Autodesk Inventor part; units mm, degrees
note: some values were not read from the file. Chosen so that the rebuilt part matches the saved one: direction of "Hole2".
(part 11 of 18)
  arc A17 (-107.2677, -34.3213) -> (-106.7778, -34.3555) centre (-106.9408, -33.1666) ccw
  line L749 (-108.0363, -21.6967) -> (-108.0269, -21.8841)
  line L750 (-107.9752, -22.9062) -> (-107.968, -23.049)
  line L751 (-107.6573, -29.1932) -> (-107.5403, -31.5077)
  line L752 (-107.4859, -32.5836) -> (-107.4515, -33.2651)
  arc A18 (-104.3538, -35.2232) -> (-104.2354, -35.2295) centre (-104.2317, -34.0295) ccw
  line L753 (-103.7167, -34.0438) -> (-103.7199, -34.1051)
  line L754 (-104.7061, -33.2435) -> (-104.7563, -34.1999)
  line L755 (-91.4937, -33.0969) -> (-91.4774, -33.1737)
  arc A19 (-88.1095, -35.5428) -> (-87.8105, -35.509) centre (-88.0934, -34.3429) ccw
  line L756 (-87.667, -33.5285) -> (-87.5609, -34.4691)
  line L757 (-88.6914, -33.6357) -> (-88.5844, -34.5846)
  arc A20 (-106.1926, -35.509) -> (-105.8936, -35.5428) centre (-105.9097, -34.3429) ccw
  line L758 (-105.3117, -33.6357) -> (-105.4187, -34.5846)
  line L759 (-106.3361, -33.5285) -> (-106.4422, -34.4691)
  line L760 (-102.5094, -33.0969) -> (-102.5257, -33.1737)
  arc A21 (-89.7677, -35.2295) -> (-89.6493, -35.2232) centre (-89.7714, -34.0295) ccw
  line L761 (-89.297, -33.2435) -> (-89.2467, -34.1999)
  line L762 (-90.2864, -34.0438) -> (-90.2831, -34.1051)
  arc A22 (-87.2253, -34.3555) -> (-86.7354, -34.3213) centre (-87.0623, -33.1666) ccw
  line L763 (-85.9668, -21.6967) -> (-85.9762, -21.8841)
  line L764 (-86.0279, -22.9062) -> (-86.0335, -23.0165)
  line L765 (-86.3442, -29.1624) -> (-86.4628, -31.5077)
  line L766 (-86.5172, -32.5836) -> (-86.5516, -33.2651)
  line L767 (-106.1877, -21.7539) -> (-106.1874, -21.795)
  line L768 (-106.1392, -29.1135) -> (-106.136, -29.6026)
  line L769 (-88.0087, -28.9946) -> (-87.8587, -30.5301)
  line L770 (-105.9944, -28.9946) -> (-106.1444, -30.5301)
  line L771 (-87.8154, -21.7539) -> (-87.8156, -21.795)
  line L772 (-87.8638, -29.1028) -> (-87.8671, -29.6026)
  ellipse E590 centre (-107.1928, -15.9924) end of major axis (-108.8923, -16.0353) minor radius 0.2846 (-108.3788, -15.8176) -> (-108.8923, -16.0353) ccw
  line L773 (-108.8884, -16.1889) -> (-108.8923, -16.0353)
  ellipse E591 centre (-86.8103, -15.9924) end of major axis (-85.1108, -16.0353) minor radius 0.2846 (-85.1108, -16.0353) -> (-85.6243, -15.8176) ccw
  line L774 (-85.1147, -16.1889) -> (-85.1108, -16.0353)
  ellipse E592 centre (-107.7158, -17.8374) end of major axis (-109.4136, -17.9232) minor radius 0.3038 (-108.6638, -17.6314) -> (-109.4136, -17.9232) ccw
  line L775 (-109.4064, -18.0666) -> (-109.4136, -17.9232)
  ellipse E593 centre (-86.2873, -17.8374) end of major axis (-84.5895, -17.9232) minor radius 0.3038 (-84.5895, -17.9232) -> (-85.3393, -17.6314) ccw
  line L776 (-84.5967, -18.0666) -> (-84.5895, -17.9232)
  ellipse E594 centre (-89.901, -14.9208) end of major axis (-88.2091, -14.7555) minor radius 0.0977 (-88.2091, -14.7555) -> (-88.7265, -14.7358) ccw
  line L777 (-88.1847, -15.005) -> (-88.2091, -14.7555)
  ellipse E595 centre (-104.1021, -14.9208) end of major axis (-105.794, -14.7555) minor radius 0.0977 (-105.2766, -14.7358) -> (-105.794, -14.7555) ccw
  line L778 (-105.8184, -15.005) -> (-105.794, -14.7555)
  ellipse E596 centre (-107.1158, -19.0477) end of major axis (-105.6163, -19.0099) minor radius 0.2511 (-106.2427, -18.8221) -> (-106.8663, -18.7939) ccw
  ellipse E597 centre (-107.1158, -19.0477) end of major axis (-105.2164, -18.9999) minor radius 0.3181 (-106.2346, -18.7443) -> (-108.1801, -18.8102) ccw
  ellipse E598 centre (-107.1854, -16.2881) end of major axis (-109.0848, -16.336) minor radius 0.3181 (-107.8873, -16.0097) -> (-109.0848, -16.336) ccw
  line L779 (-109.05, -17.7146) -> (-109.0848, -16.336)
  ellipse E599 centre (-89.5506, -19.9696) end of major axis (-87.6609, -19.7717) minor radius 0.0812 (-87.8191, -19.8213) -> (-87.8776, -19.7568) ccw
  ellipse E600 centre (-89.8419, -17.1874) end of major axis (-87.9523, -16.9895) minor radius 0.0812 (-88.063, -16.9739) -> (-88.4635, -16.9874) ccw
  line L780 (-87.6609, -19.7717) -> (-87.8661, -17.8124)
  ellipse E601 centre (-104.4525, -19.9696) end of major axis (-106.3422, -19.7717) minor radius 0.0812 (-106.1255, -19.7568) -> (-106.184, -19.8213) ccw
  ellipse E602 centre (-104.1611, -17.1874) end of major axis (-106.0508, -16.9895) minor radius 0.0812 (-105.5396, -16.9874) -> (-105.9401, -16.9739) ccw
  line L781 (-106.3422, -19.7717) -> (-106.137, -17.8124)
  ellipse E603 centre (-86.8872, -19.0477) end of major axis (-85.3877, -19.0855) minor radius 0.2511 (-87.1368, -18.7939) -> (-87.7604, -18.8221) ccw
  ellipse E604 centre (-86.8872, -19.0477) end of major axis (-84.9878, -19.0956) minor radius 0.3181 (-85.823, -18.8102) -> (-87.7685, -18.7443) ccw
  ellipse E605 centre (-86.8177, -16.2881) end of major axis (-84.9183, -16.336) minor radius 0.3181 (-84.9183, -16.336) -> (-86.1158, -16.0097) ccw
  line L782 (-84.953, -17.7146) -> (-84.9183, -16.336)
  ellipse E606 centre (-107.5618, -20.8836) end of major axis (-109.0599, -20.9593) minor radius 0.2681 (-106.281, -20.6817) -> (-108.7521, -21.1048) ccw
  ellipse E607 centre (-107.5618, -20.8836) end of major axis (-109.4594, -20.9795) minor radius 0.3396 (-106.2686, -20.5715) -> (-108.747, -21.2071) ccw
  ellipse E608 centre (-107.7009, -18.1322) end of major axis (-109.5985, -18.2281) minor radius 0.3396 (-108.2162, -17.8302) -> (-109.5985, -18.2281) ccw
  line L783 (-109.4594, -20.9795) -> (-109.5985, -18.2281)
  ellipse E609 centre (-89.4939, -21.9244) end of major axis (-87.6059, -21.7115) minor radius 0.0405 (-87.9052, -21.7673) -> (-87.9103, -21.7237) ccw
  ellipse E610 centre (-89.8077, -19.1427) end of major axis (-87.9196, -18.9298) minor radius 0.0405 (-87.9691, -18.9262) -> (-88.2351, -18.9429) ccw
  line L784 (-87.6059, -21.7115) -> (-87.8249, -19.77)
  ellipse E611 centre (-104.5091, -21.9244) end of major axis (-106.3972, -21.7115) minor radius 0.0405 (-106.0928, -21.7237) -> (-106.0979, -21.7673) ccw
  ellipse E612 centre (-104.1954, -19.1427) end of major axis (-106.0834, -18.9298) minor radius 0.0405 (-105.768, -18.9429) -> (-106.034, -18.9262) ccw
  line L785 (-106.3972, -21.7115) -> (-106.1782, -19.77)
  ellipse E613 centre (-86.4413, -20.8836) end of major axis (-84.9432, -20.9593) minor radius 0.2681 (-85.251, -21.1048) -> (-87.7221, -20.6817) ccw
  ellipse E614 centre (-86.4413, -20.8836) end of major axis (-84.5437, -20.9795) minor radius 0.3396 (-85.2561, -21.2071) -> (-87.7345, -20.5715) ccw
  ellipse E615 centre (-86.3022, -18.1322) end of major axis (-84.4046, -18.2281) minor radius 0.3396 (-84.4046, -18.2281) -> (-85.7868, -17.8302) ccw
  line L786 (-84.5437, -20.9795) -> (-84.4046, -18.2281)
  ellipse E616 centre (-106.7329, -17.1735) end of major axis (-105.2329, -17.1637) minor radius 0.2359 (-106.2093, -16.9491) -> (-106.2264, -16.9483) ccw
  ellipse E617 centre (-106.7329, -17.1735) end of major axis (-104.8329, -17.161) minor radius 0.2988 (-106.2028, -16.8832) -> (-107.8731, -16.9419) ccw
  ellipse E618 centre (-106.7511, -14.4084) end of major axis (-108.6511, -14.421) minor radius 0.2988 (-108.5711, -14.3344) -> (-108.6511, -14.421) ccw
  line L787 (-108.6415, -15.8791) -> (-108.6511, -14.421)
  ellipse E619 centre (-89.6001, -18.001) end of major axis (-87.7091, -17.8163) minor radius 0.1092 (-87.8596, -17.8744) -> (-87.9801, -17.7867) ccw
  ellipse E620 centre (-89.8719, -15.2189) end of major axis (-87.9809, -15.0341) minor radius 0.1092 (-87.9809, -15.0341) -> (-88.6935, -15.0183) ccw
  line L788 (-87.7091, -17.8163) -> (-87.9809, -15.0341)
  ellipse E621 centre (-104.403, -18.001) end of major axis (-106.294, -17.8163) minor radius 0.1092 (-106.0229, -17.7867) -> (-106.1435, -17.8744) ccw
  ellipse E622 centre (-104.1312, -15.2189) end of major axis (-106.0222, -15.0341) minor radius 0.1092 (-105.3096, -15.0183) -> (-106.0222, -15.0341) ccw
  line L789 (-106.294, -17.8163) -> (-106.0222, -15.0341)
  ellipse E623 centre (-87.2702, -17.1735) end of major axis (-85.7702, -17.1834) minor radius 0.2359 (-87.7766, -16.9483) -> (-87.7938, -16.9491) ccw
  ellipse E624 centre (-87.2702, -17.1735) end of major axis (-85.3702, -17.1861) minor radius 0.2988 (-86.1299, -16.9419) -> (-87.8003, -16.8832) ccw
  ellipse E625 centre (-87.252, -14.4084) end of major axis (-85.352, -14.421) minor radius 0.2988 (-85.352, -14.421) -> (-85.432, -14.3344) ccw
  line L790 (-85.3616, -15.8791) -> (-85.352, -14.421)
  line L791 (-105.7463, -23.3854) -> (-105.7298, -23.4858)
  line L792 (-105.7134, -23.5857) -> (-104.5188, -30.8738)
  line L793 (-100.5406, -31.29) -> (-99.6819, -29.0825)
  line L794 (-100.5406, -31.29) -> (-100.5406, -31.29)
  line L795 (-105.1682, -17.8599) -> (-105.548, -21.4907)
  line L796 (-105.7458, -23.3806) -> (-105.7463, -23.3854)
  line L797 (-105.1682, -17.8599) -> (-105.2441, -18.5851)
  line L798 (-100.6125, -31.2825) -> (-100.5406, -31.29)
  line L799 (-104.5188, -30.8738) -> (-104.0963, -30.918)
  line L800 (-102.4378, -31.0915) -> (-100.5406, -31.29)
  ellipse E626 centre (-105.1683, -17.8599) end of major axis (-105.2212, -18.3652) minor radius 0.0001 (-105.1682, -17.8599) -> (-105.1438, -17.6266) ccw
  ellipse E627 centre (-105.1683, -17.8599) end of major axis (-105.2741, -18.8704) minor radius 0.0002 (-105.1682, -17.8599) -> (-105.1194, -17.3933) ccw
  ellipse E628 centre (-104.4874, -11.3464) end of major axis (-104.3817, -10.336) minor radius 0.0002 (-104.4384, -10.8798) -> (-104.3817, -10.336) ccw
  ellipse E629 centre (-104.4874, -11.3464) end of major axis (-104.4345, -10.8412) minor radius 0.0001 (-104.4629, -11.1131) -> (-104.4345, -10.8412) ccw
  line L801 (-104.3817, -10.336) -> (-104.0713, -10.3684)
  line L802 (-105.1438, -17.6266) -> (-104.4629, -11.1131)
  line L803 (-105.1194, -17.3933) -> (-104.4384, -10.8798)
  line L804 (-104.3818, -10.336) -> (-105.3769, -10.2321)
  line L805 (-105.4298, -10.7374) -> (-105.3769, -10.2321)
  line L806 (-105.4298, -10.7374) -> (-104.4347, -10.8413)
  line L807 (-104.3818, -10.336) -> (-104.4347, -10.8413)
  line L808 (-105.3769, -10.2321) -> (-105.377, -10.2322)
  line L809 (-104.4347, -10.8413) -> (-104.4345, -10.8412)
  line L810 (-104.3817, -10.336) -> (-104.3818, -10.336)
  line L811 (-101.0015, -16.9313) -> (-101.0015, -17.6075)
  line L812 (-93.0015, -16.9313) -> (-93.0015, -17.6075)
  line L813 (-101.0015, -16.9313) -> (-101.0015, -16.4767)
  line L814 (-93.0015, -16.9313) -> (-93.0015, -16.4767)
  line L815 (-101.0015, -16.4767) -> (-101.0015, -16.0045)
  line L816 (-93.0015, -16.0045) -> (-93.0015, -16.4767)
  line L817 (-92.68, -10.0775) -> (-93.0015, -9.9718)
  line L818 (-93.0015, -10.4771) -> (-92.7422, -10.5624)
  line L819 (-101.0015, -9.9718) -> (-101.323, -10.0775)
  line L820 (-101.2609, -10.5624) -> (-101.0015, -10.4771)
  line L821 (-93.4625, -31.29) -> (-93.4624, -31.29)
  line L822 (-94.3212, -29.0825) -> (-93.4625, -31.29)
  line L823 (-89.4842, -30.8738) -> (-88.2896, -23.5857)
  line L824 (-88.2733, -23.4858) -> (-88.2568, -23.3854)
  line L825 (-88.759, -18.5851) -> (-88.8348, -17.8599)
  line L826 (-88.8349, -17.8599) -> (-88.455, -21.4907)
  line L827 (-88.2573, -23.3806) -> (-88.2568, -23.3854)
  line L828 (-93.4624, -31.29) -> (-93.3906, -31.2825)
  line L829 (-93.4625, -31.29) -> (-91.5653, -31.0915)
  line L830 (-89.9068, -30.918) -> (-89.4842, -30.8738)
  ellipse E630 centre (-88.8348, -17.8599) end of major axis (-88.8876, -17.3547) minor radius 0.0001 (-88.8592, -17.6266) -> (-88.8348, -17.8599) ccw
  ellipse E631 centre (-88.8348, -17.8599) end of major axis (-88.729, -18.8704) minor radius 0.0002 (-88.8837, -17.3933) -> (-88.8349, -17.8599) ccw
  ellipse E632 centre (-89.5157, -11.3464) end of major axis (-89.6214, -10.336) minor radius 0.0002 (-89.6214, -10.336) -> (-89.5647, -10.8798) ccw
  ellipse E633 centre (-89.5157, -11.3464) end of major axis (-89.5686, -10.8412) minor radius 0.0001 (-89.5686, -10.8412) -> (-89.5402, -11.1131) ccw
  line L831 (-89.9318, -10.3684) -> (-89.6214, -10.336)
  line L832 (-88.8592, -17.6266) -> (-89.5402, -11.1131)
  line L833 (-89.5647, -10.8798) -> (-88.8837, -17.3933)
  line L834 (-88.6262, -10.2321) -> (-89.6213, -10.336)
  line L835 (-89.5684, -10.8413) -> (-89.6213, -10.336)
  line L836 (-89.5684, -10.8413) -> (-88.5733, -10.7374)
  line L837 (-88.5733, -10.7374) -> (-88.6262, -10.2321)
  line L838 (-88.6261, -10.2322) -> (-88.6262, -10.2321)
  line L839 (-89.6213, -10.336) -> (-89.6214, -10.336)
  line L840 (-89.5686, -10.8412) -> (-89.5684, -10.8413)
  line L841 (-99.9835, -29.8578) -> (-99.0015, -33.4516)
  line L842 (-95.0015, -33.4516) -> (-94.0196, -29.8578)
  line L843 (-99.0015, -33.4516) -> (-95.0015, -33.4516)
  line L844 (-99.377, -33.13) -> (-99.0015, -34.4948)
  line L845 (-95.0015, -34.4948) -> (-94.6287, -33.1394)
  line L846 (-99.0015, -34.4948) -> (-95.0015, -34.4948)
  line L847 (-105.369, -32.7627) -> (-106.506, -25.2601)
  line L848 (-105.3689, -32.7627) -> (-105.369, -32.7627)
  line L849 (-106.506, -25.2601) -> (-105.3689, -32.7627)
  line L850 (-106.506, -25.2601) -> (-106.506, -25.2601)
  line L851 (-101.396, -33.2269) -> (-100.6125, -31.2825)
  line L852 (-101.396, -33.2269) -> (-101.396, -33.2269)
  line L853 (-105.8612, -19.7419) -> (-106.506, -25.2601)
  line L854 (-105.8613, -19.742) -> (-106.506, -25.2601)
  line L855 (-105.369, -32.7627) -> (-101.396, -33.2269)
  line L856 (-105.3689, -32.7627) -> (-101.396, -33.2269)
  ellipse E634 centre (-105.8613, -19.742) end of major axis (-105.9203, -20.2465) minor radius 0 (-105.8613, -19.742) -> (-105.8341, -19.509) ccw
  ellipse E635 centre (-105.8613, -19.742) end of major axis (-105.9792, -20.7511) minor radius 0.0001 (-105.8612, -19.7419) -> (-105.8068, -19.276) ccw
  ellipse E636 centre (-105.1017, -13.2371) end of major axis (-104.9838, -12.228) minor radius 0.0001 (-105.0471, -12.7711) -> (-104.9838, -12.228) ccw
  ellipse E637 centre (-105.1017, -13.2371) end of major axis (-105.0427, -12.7326) minor radius 0 (-105.0744, -13.0041) -> (-105.0427, -12.7326) ccw
  line L857 (-104.9838, -12.228) -> (-104.5843, -12.2747)
  line L858 (-105.8341, -19.509) -> (-105.0744, -13.0041)
  line L859 (-105.8068, -19.276) -> (-105.0471, -12.7711)
  line L860 (-104.9839, -12.228) -> (-105.9774, -12.1121)
  line L861 (-106.0364, -12.6167) -> (-105.9774, -12.1121)
  line L862 (-106.0364, -12.6167) -> (-105.0428, -12.7326)
  line L863 (-104.9839, -12.228) -> (-105.0428, -12.7326)
  line L864 (-105.9774, -12.1121) -> (-105.9775, -12.1121)
  line L865 (-105.0428, -12.7326) -> (-105.0427, -12.7326)
  line L866 (-104.9838, -12.228) -> (-104.9839, -12.228)
  line L867 (-99.0015, -31.5559) -> (-101.0015, -24.2852)
  line L868 (-99.0015, -31.497) -> (-99.0015, -31.5559)
  line L869 (-101.0015, -24.2263) -> (-99.0015, -31.497)
  line L870 (-101.0015, -24.2852) -> (-101.0015, -24.2263)
  line L871 (-93.0015, -24.2852) -> (-95.0015, -31.5559)
  line L872 (-93.0015, -24.2263) -> (-93.0015, -24.2852)
  line L873 (-95.0015, -31.497) -> (-93.0015, -24.2263)
  line L874 (-95.0015, -31.5559) -> (-95.0015, -31.497)
  line L875 (-101.0015, -18.7081) -> (-101.0015, -24.2263)
  line L876 (-93.0015, -18.7081) -> (-93.0015, -24.2263)
  line L877 (-99.0015, -31.5559) -> (-95.0015, -31.5559)
  line L878 (-99.0015, -31.497) -> (-95.0015, -31.497)
  line L879 (-101.0015, -18.7081) -> (-101.0015, -18.2554)
  line L880 (-93.0015, -18.7081) -> (-93.0015, -18.2554)
  line L881 (-101.0015, -18.2554) -> (-101.0015, -17.6075)
  line L882 (-93.0015, -17.6075) -> (-93.0015, -18.2554)
  line L883 (-92.789, -11.9006) -> (-93.0015, -11.8228)
  line L884 (-93.0015, -12.3273) -> (-92.8489, -12.3832)
  line L885 (-101.0015, -11.8228) -> (-101.2141, -11.9006)
  line L886 (-101.1541, -12.3832) -> (-101.0015, -12.3273)
  line L887 (-92.6071, -33.2269) -> (-92.6071, -33.2269)
  line L888 (-93.3906, -31.2825) -> (-92.6071, -33.2269)
  line L889 (-87.4971, -25.2601) -> (-88.6341, -32.7627)
  line L890 (-87.4971, -25.2601) -> (-87.4971, -25.2601)
  line L891 (-88.6341, -32.7627) -> (-87.4971, -25.2601)
  line L892 (-88.6341, -32.7627) -> (-88.6341, -32.7627)
  line L893 (-87.4971, -25.2601) -> (-88.1418, -19.742)
  line L894 (-88.1419, -19.7419) -> (-87.4971, -25.2601)
  line L895 (-92.6071, -33.2269) -> (-88.6341, -32.7627)
  line L896 (-92.6071, -33.2269) -> (-88.6341, -32.7627)
  ellipse E638 centre (-88.1417, -19.742) end of major axis (-88.2007, -19.2374) minor radius 0 (-88.169, -19.509) -> (-88.1418, -19.742) ccw
  ellipse E639 centre (-88.1417, -19.742) end of major axis (-88.0238, -20.7511) minor radius 0.0001 (-88.1963, -19.276) -> (-88.1419, -19.7419) ccw
  ellipse E640 centre (-88.9014, -13.2371) end of major axis (-89.0193, -12.228) minor radius 0.0001 (-89.0193, -12.228) -> (-88.956, -12.7711) ccw
  ellipse E641 centre (-88.9014, -13.2371) end of major axis (-88.9604, -12.7326) minor radius 0 (-88.9604, -12.7326) -> (-88.9287, -13.0041) ccw
  line L897 (-89.4187, -12.2747) -> (-89.0193, -12.228)
  line L898 (-88.169, -19.509) -> (-88.9287, -13.0041)
  line L899 (-88.956, -12.7711) -> (-88.1963, -19.276)
  line L900 (-88.0257, -12.1121) -> (-89.0192, -12.228)
  line L901 (-88.9603, -12.7326) -> (-89.0192, -12.228)
  line L902 (-88.9603, -12.7326) -> (-87.9667, -12.6167)
  line L903 (-87.9667, -12.6167) -> (-88.0257, -12.1121)
  line L904 (-88.0256, -12.1121) -> (-88.0257, -12.1121)
  line L905 (-89.0192, -12.228) -> (-89.0193, -12.228)
  line L906 (-88.9604, -12.7326) -> (-88.9603, -12.7326)
  line L907 (-104.6002, -15.9516) -> (-104.7812, -17.861)
  line L908 (-104.6003, -15.9516) -> (-104.6693, -16.6796)
  ellipse E642 centre (-104.6003, -15.9516) end of major axis (-104.6482, -16.4573) minor radius 0 (-104.6003, -15.9516) -> (-104.5781, -15.718) ccw
  ellipse E643 centre (-104.6003, -15.9516) end of major axis (-104.6962, -16.963) minor radius 0.0001 (-104.6002, -15.9516) -> (-104.556, -15.4845) ccw
  ellipse E644 centre (-103.9825, -9.4316) end of major axis (-103.8867, -8.4201) minor radius 0.0001 (-103.9382, -8.9645) -> (-103.8867, -8.4201) ccw
  ellipse E645 centre (-103.9825, -9.4316) end of major axis (-103.9346, -8.9259) minor radius 0 (-103.9604, -9.1981) -> (-103.9346, -8.9259) ccw
  line L909 (-103.8867, -8.4201) -> (-101.6065, -8.6362)
  line L910 (-104.5781, -15.718) -> (-103.9604, -9.1981)
  line L911 (-104.556, -15.4845) -> (-103.9382, -8.9645)
  line L912 (-103.8867, -8.4201) -> (-104.8825, -8.3258)
  line L913 (-104.9304, -8.8315) -> (-104.8825, -8.3258)
  line L914 (-104.9304, -8.8315) -> (-103.9347, -8.9259)
  line L915 (-103.8867, -8.4201) -> (-103.9347, -8.9259)
  line L916 (-104.8825, -8.3258) -> (-104.8826, -8.3258)
  line L917 (-103.9347, -8.9259) -> (-103.9346, -8.9259)
  line L918 (-103.8867, -8.4201) -> (-103.8867, -8.4201)
  line L919 (-101.0015, -15.11) -> (-101.0015, -16.0045)
  line L920 (-93.0015, -15.11) -> (-93.0015, -16.0045)
  line L921 (-101.0015, -15.11) -> (-101.0015, -14.6537)
  line L922 (-93.0015, -15.11) -> (-93.0015, -14.6537)
  line L923 (-93.0015, -8.4553) -> (-93.0015, -7.9913)
  line L924 (-101.0015, -7.9913) -> (-101.0015, -8.4553)
  line L925 (-101.0015, -7.9913) -> (-93.0015, -7.9913)
  line L926 (-101.0015, -14.6537) -> (-101.0015, -8.4553)
  line L927 (-93.0015, -8.4553) -> (-93.0015, -14.6537)
  line L928 (-92.0015, -8.3883) -> (-93.0015, -8.0902)
  line L929 (-93.0015, -8.5959) -> (-92.5247, -8.7381)
  line L930 (-92.0015, -8.5988) -> (-92.0015, -8.3883)
  line L931 (-101.0015, -8.0902) -> (-102.0015, -8.3883)
  line L932 (-102.0015, -8.5988) -> (-102.0015, -8.3883)
  line L933 (-101.4783, -8.7381) -> (-101.0015, -8.5959)
  line L934 (-89.3338, -16.6796) -> (-89.4028, -15.9516)
  line L935 (-89.4029, -15.9516) -> (-89.2219, -17.861)
  ellipse E646 centre (-89.4028, -15.9516) end of major axis (-89.4507, -15.4458) minor radius 0 (-89.425, -15.718) -> (-89.4028, -15.9516) ccw
  ellipse E647 centre (-89.4028, -15.9516) end of major axis (-89.3069, -16.963) minor radius 0.0001 (-89.4471, -15.4845) -> (-89.4029, -15.9516) ccw
  ellipse E648 centre (-90.0205, -9.4316) end of major axis (-90.1164, -8.4201) minor radius 0.0001 (-90.1164, -8.4201) -> (-90.0649, -8.9645) ccw
  ellipse E649 centre (-90.0205, -9.4316) end of major axis (-90.0685, -8.9259) minor radius 0 (-90.0685, -8.9259) -> (-90.0427, -9.1981) ccw
  line L936 (-92.3966, -8.6362) -> (-90.1164, -8.4201)
  line L937 (-89.425, -15.718) -> (-90.0427, -9.1981)
  line L938 (-90.0649, -8.9645) -> (-89.4471, -15.4845)
  line L939 (-89.1206, -8.3258) -> (-90.1163, -8.4201)
  line L940 (-90.0684, -8.9259) -> (-90.1163, -8.4201)
  line L941 (-90.0684, -8.9259) -> (-89.0726, -8.8315)
  line L942 (-89.0726, -8.8315) -> (-89.1206, -8.3258)
  line L943 (-89.1205, -8.3258) -> (-89.1206, -8.3258)
  line L944 (-90.1163, -8.4201) -> (-90.1164, -8.4201)
  line L945 (-90.0685, -8.9259) -> (-90.0684, -8.9259)
  line L946 (-104.7832, -19.61) -> (-104.7624, -19.4112)
  line L947 (-104.7622, -19.4111) -> (-104.783, -19.6101)
  line L948 (-104.7624, -19.4112) -> (-104.7622, -19.4111)
  line L949 (-105.0316, -19.584) -> (-105.0318, -19.5841)
  line L950 (-104.783, -19.6101) -> (-105.0316, -19.584)
  line L951 (-103.7884, -19.7141) -> (-103.7676, -19.5152)
  line L952 (-103.5398, -19.7401) -> (-103.7884, -19.7141)
  line L953 (-103.7377, -21.6299) -> (-103.9861, -21.6039)
  line L954 (-103.7375, -21.6298) -> (-103.7377, -21.6299)
  line L955 (-104.0069, -21.8027) -> (-103.9861, -21.6038)
  line L956 (-103.9861, -21.6038) -> (-103.7375, -21.6298)
  line L957 (-104.0072, -21.8028) -> (-104.0069, -21.8027)
  line L958 (-104.0072, -21.8028) -> (-104.2713, -21.7752)
  line L959 (-105.2143, -21.3283) -> (-105.0318, -19.5841)
  line L960 (-104.7622, -19.4111) -> (-103.7676, -19.5152)
  line L961 (-103.5398, -19.7401) -> (-103.7375, -21.6298)
  line L962 (-105.2293, -21.4737) -> (-105.0316, -19.584)
  line L963 (-104.0069, -21.8027) -> (-105.0015, -21.6987)
  line L964 (-105.2293, -21.4737) -> (-104.9807, -21.4997)
  line L965 (-104.9807, -21.4997) -> (-105.0015, -21.6987)
  line L966 (-103.8092, -19.913) -> (-103.9653, -21.4049)
  line L967 (-103.9653, -21.4049) -> (-104.9599, -21.3008)
  line L968 (-104.9599, -21.3008) -> (-104.8038, -19.809)
  line L969 (-104.8038, -19.809) -> (-103.8092, -19.913)
  line L970 (-104.1225, -21.2112) -> (-104.0031, -20.0701)
  line L971 (-103.9653, -21.4049) -> (-104.1225, -21.2112)
  line L972 (-103.8092, -19.913) -> (-104.0031, -20.0701)
  line L973 (-104.0031, -20.0701) -> (-104.6469, -20.0027)
  line L974 (-104.8038, -19.809) -> (-104.6469, -20.0027)
  line L975 (-104.6469, -20.0027) -> (-104.7663, -21.1439)
  line L976 (-104.9599, -21.3008) -> (-104.7663, -21.1439)
  line L977 (-104.7663, -21.1439) -> (-104.1225, -21.2112)
  circle A23 centre (-104.3574, -20.3465) radius 0.1
  line L978 (-104.5235, -20.4919) -> (-104.4898, -20.1698)
  line L979 (-104.4898, -20.1698) -> (-104.4898, -20.1698)
  line L980 (-104.5235, -20.4919) -> (-104.4898, -20.1698)
  line L981 (-104.5235, -20.4919) -> (-104.5235, -20.4919)
  line L982 (-104.4898, -20.1698) -> (-104.1914, -20.2011)
  line L983 (-104.1914, -20.2011) -> (-104.2251, -20.5231)
  line L984 (-104.2251, -20.5231) -> (-104.2251, -20.5231)
  line L985 (-104.2251, -20.5231) -> (-104.5235, -20.4919)
  line L986 (-104.2251, -20.5231) -> (-104.5235, -20.4919)
  line L987 (-103.3965, -30.2371) -> (-103.5954, -30.2163)
  line L988 (-103.3963, -30.237) -> (-103.3965, -30.2371)
  line L989 (-103.5952, -30.2162) -> (-103.3963, -30.237)
  line L990 (-103.5954, -30.2163) -> (-103.5952, -30.2162)
  line L991 (-103.4225, -30.4858) -> (-103.3965, -30.2371)
  line L992 (-103.4223, -30.4857) -> (-103.4225, -30.4858)
  line L993 (-103.3963, -30.237) -> (-103.4223, -30.4857)
  line L994 (-103.2924, -29.2424) -> (-103.2664, -28.9939)
  line L995 (-103.4911, -29.2217) -> (-103.4913, -29.2217)
  line L996 (-103.2922, -29.2425) -> (-103.4911, -29.2217)
  line L997 (-103.2662, -28.9938) -> (-103.2922, -29.2425)
  line L998 (-103.2664, -28.9939) -> (-103.2662, -28.9938)
  line L999 (-103.5954, -30.2163) -> (-103.4913, -29.2217)
  line L1000 (-101.5328, -30.6835) -> (-103.4225, -30.4858)
  line L1001 (-103.5952, -30.2162) -> (-103.4911, -29.2217)
  line L1002 (-103.2662, -28.9938) -> (-101.3765, -29.1915)
  line L1003 (-101.5326, -30.6834) -> (-103.4223, -30.4857)
  line L1004 (-101.2036, -29.461) -> (-101.3077, -30.4556)
  line L1005 (-101.3079, -30.4556) -> (-101.5066, -30.4349)
  line L1006 (-101.5326, -30.6834) -> (-101.5066, -30.4348)
  line L1007 (-101.5066, -30.4348) -> (-101.3077, -30.4556)
  line L1008 (-101.3077, -30.4556) -> (-101.3079, -30.4556)
  line L1009 (-101.5328, -30.6835) -> (-101.5326, -30.6834)
  line L1010 (-101.2036, -29.461) -> (-101.4025, -29.4402)
  line L1011 (-101.4025, -29.4402) -> (-101.3765, -29.1915)
  line L1012 (-103.0933, -29.2633) -> (-101.6014, -29.4194)
  line L1013 (-101.6014, -29.4194) -> (-101.7055, -30.4139)
  line L1014 (-101.7055, -30.4139) -> (-103.1974, -30.2579)
  line L1015 (-103.1974, -30.2579) -> (-103.0933, -29.2633)
  line L1016 (-101.7953, -29.5764) -> (-102.9364, -29.4571)
  line L1017 (-101.6014, -29.4194) -> (-101.7953, -29.5764)
  line L1018 (-103.0933, -29.2633) -> (-102.9364, -29.4571)
  line L1019 (-102.9364, -29.4571) -> (-103.0038, -30.1009)
  line L1020 (-103.1974, -30.2579) -> (-103.0038, -30.1009)
  line L1021 (-103.0038, -30.1009) -> (-101.8627, -30.2203)
  line L1022 (-101.7055, -30.4139) -> (-101.8627, -30.2203)
  line L1023 (-101.8627, -30.2203) -> (-101.7953, -29.5764)
  circle A24 centre (-102.66, -29.8114) radius 0.1
  line L1024 (-102.5146, -29.9774) -> (-102.8367, -29.9437)
  line L1025 (-102.8367, -29.9438) -> (-102.8367, -29.9437)
  line L1026 (-102.5146, -29.9774) -> (-102.8367, -29.9438)
  line L1027 (-102.5146, -29.9774) -> (-102.5146, -29.9774)
  line L1028 (-102.8367, -29.9437) -> (-102.8054, -29.6454)
  line L1029 (-102.8055, -29.6454) -> (-102.8054, -29.6454)
  line L1030 (-102.8367, -29.9438) -> (-102.8055, -29.6454)
  line L1031 (-102.8054, -29.6454) -> (-102.4834, -29.6791)
  line L1032 (-102.4834, -29.6791) -> (-102.5146, -29.9774)
  line L1033 (-100.4365, -18.2782) -> (-100.4365, -18.4771)
  line L1034 (-100.4365, -18.4771) -> (-100.6865, -18.4771)
  line L1035 (-99.4365, -18.4771) -> (-99.4365, -18.2782)
  line L1036 (-99.1865, -18.4771) -> (-99.4365, -18.4771)
  line L1037 (-100.4365, -18.2782) -> (-99.4365, -18.2782)
  line L1038 (-99.1865, -18.4771) -> (-99.1865, -20.235)
  line L1039 (-100.6865, -20.235) -> (-100.6865, -18.4771)
  line L1040 (-99.4365, -18.676) -> (-99.4365, -20.0364)
  line L1041 (-100.4365, -20.0364) -> (-100.4365, -18.676)
  line L1042 (-100.4365, -18.676) -> (-99.4365, -18.676)
  line L1043 (-99.4365, -18.676) -> (-99.5965, -18.9295)
  line L1044 (-100.4365, -18.676) -> (-100.2766, -18.9295)
  ellipse E650 centre (-99.9365, -19.2395) end of major axis (-99.8365, -19.2395) minor radius 0.0995
  ellipse E651 centre (-99.9365, -19.2447) end of major axis (-99.8365, -19.2447) minor radius 0.0995 (-100.0365, -19.2447) -> (-99.8365, -19.2447) ccw
  line L1045 (-100.0365, -19.2447) -> (-100.0365, -19.2395)
  line L1046 (-99.8365, -19.2447) -> (-99.8365, -19.2395)
  line L1047 (-100.0865, -19.4057) -> (-100.0865, -19.0837)
  line L1048 (-100.0865, -19.4163) -> (-100.0865, -19.4057)
  line L1049 (-100.0865, -19.0837) -> (-99.7865, -19.0837)
  line L1050 (-99.7865, -19.0837) -> (-99.7865, -19.4057)
  line L1051 (-99.7865, -19.4163) -> (-99.7865, -19.4057)
  line L1052 (-99.7865, -19.4057) -> (-100.0865, -19.4057)
  line L1053 (-98.1515, -28.8455) -> (-97.9515, -28.8455)
  line L1054 (-98.1515, -28.9274) -> (-98.1515, -28.8455)
  line L1055 (-97.9515, -29.0941) -> (-97.9515, -29.1757)
  line L1056 (-97.9515, -28.8455) -> (-97.9515, -29.0941)
  line L1057 (-97.9515, -27.8509) -> (-98.1515, -27.8509)
  line L1058 (-97.9515, -27.6023) -> (-97.9515, -27.8509)
  line L1059 (-98.1515, -28.8455) -> (-98.1515, -27.8509)
  line L1060 (-97.9515, -27.6023) -> (-96.0515, -27.6023)
  line L1061 (-96.0515, -29.0941) -> (-97.9515, -29.0941)
  line L1062 (-95.8515, -27.8509) -> (-95.8515, -28.8455)
  line L1063 (-96.0515, -29.0941) -> (-96.0515, -28.8455)
  line L1064 (-96.0515, -28.8455) -> (-95.8515, -28.8455)
  line L1065 (-95.8515, -28.8455) -> (-95.8515, -28.9274)
  line L1066 (-96.0515, -29.1757) -> (-96.0515, -29.0941)
  line L1067 (-95.8515, -27.8509) -> (-96.0515, -27.8509)
  line L1068 (-96.0515, -27.8509) -> (-96.0515, -27.6023)
  line L1069 (-97.7515, -27.8509) -> (-96.2515, -27.8509)
  line L1070 (-96.2515, -27.8509) -> (-96.2515, -28.8455)
  line L1071 (-96.2515, -28.8455) -> (-97.7515, -28.8455)
  line L1072 (-97.7515, -28.8455) -> (-97.7515, -27.8509)
  line L1073 (-96.2515, -27.8509) -> (-96.3922, -28.0738)
  line L1074 (-97.7515, -27.8509) -> (-97.6109, -28.0738)
  line L1075 (-97.7515, -28.8455) -> (-97.6124, -28.7892)
  line L1076 (-96.2515, -28.8455) -> (-96.3906, -28.7892)
  ellipse E652 centre (-97.2635, -28.4263) end of major axis (-97.1635, -28.4263) minor radius 0.0995
  line L1077 (-97.3635, -28.4307) -> (-97.3635, -28.4263)
  line L1078 (-97.1635, -28.4307) -> (-97.1635, -28.4263)
  line L1079 (-92.4965, -30.4349) -> (-92.6952, -30.4556)
  line L1080 (-92.6954, -30.4556) -> (-92.4965, -30.4348)
  line L1081 (-92.6952, -30.4556) -> (-92.6954, -30.4556)
  line L1082 (-92.4705, -30.6834) -> (-92.4703, -30.6835)
  line L1083 (-92.4965, -30.4348) -> (-92.4705, -30.6834)
  line L1084 (-92.6006, -29.4402) -> (-92.7995, -29.461)
  line L1085 (-92.6266, -29.1915) -> (-92.6006, -29.4402)
  line L1086 (-90.7367, -28.9939) -> (-90.7107, -29.2424)
  line L1087 (-90.7369, -28.9938) -> (-90.7367, -28.9939)
  line L1088 (-90.512, -29.2217) -> (-90.7109, -29.2425)
  line L1089 (-90.7109, -29.2425) -> (-90.7369, -28.9938)
  line L1090 (-90.5117, -29.2217) -> (-90.512, -29.2217)
  line L1091 (-90.5117, -29.2217) -> (-90.4077, -30.2163)
  line L1092 (-90.5806, -30.4858) -> (-92.4703, -30.6835)
  line L1093 (-92.6954, -30.4556) -> (-92.7995, -29.461)
  line L1094 (-92.6266, -29.1915) -> (-90.7369, -28.9938)
  line L1095 (-90.5808, -30.4857) -> (-92.4705, -30.6834)
  line L1096 (-90.512, -29.2217) -> (-90.4079, -30.2162)
  line L1097 (-90.4077, -30.2163) -> (-90.6066, -30.2371)
  line L1098 (-90.6066, -30.2371) -> (-90.5806, -30.4858)
  line L1099 (-90.5808, -30.4857) -> (-90.6068, -30.237)
  line L1100 (-90.6068, -30.237) -> (-90.4079, -30.2162)
  line L1101 (-90.4079, -30.2162) -> (-90.4077, -30.2163)
  line L1102 (-90.6068, -30.237) -> (-90.6066, -30.2371)
  line L1103 (-90.5806, -30.4858) -> (-90.5808, -30.4857)
  line L1104 (-92.4016, -29.4194) -> (-90.9098, -29.2633)
  line L1105 (-90.9098, -29.2633) -> (-90.8057, -30.2579)
  line L1106 (-90.8057, -30.2579) -> (-92.2976, -30.4139)
  line L1107 (-92.2976, -30.4139) -> (-92.4016, -29.4194)
  line L1108 (-91.0666, -29.4571) -> (-92.2078, -29.5764)
  line L1109 (-90.9098, -29.2633) -> (-91.0666, -29.4571)
  line L1110 (-92.4016, -29.4194) -> (-92.2078, -29.5764)
  line L1111 (-92.2078, -29.5764) -> (-92.1404, -30.2203)
  line L1112 (-92.2976, -30.4139) -> (-92.1404, -30.2203)
  line L1113 (-92.1404, -30.2203) -> (-90.9993, -30.1009)
  line L1114 (-90.8057, -30.2579) -> (-90.9993, -30.1009)
  line L1115 (-90.9993, -30.1009) -> (-91.0666, -29.4571)
  circle A25 centre (-91.8641, -29.8659) radius 0.1
  line L1116 (-91.6874, -29.9982) -> (-92.0095, -30.0319)
  line L1117 (-92.0094, -30.032) -> (-92.0095, -30.0319)
  line L1118 (-91.6874, -29.9983) -> (-92.0094, -30.032)
  line L1119 (-91.6874, -29.9983) -> (-91.6874, -29.9982)
  line L1120 (-92.0095, -30.0319) -> (-92.0407, -29.7336)
  line L1121 (-92.0407, -29.7336) -> (-91.7186, -29.6999)
  line L1122 (-91.7186, -29.6999) -> (-91.7186, -29.6999)
  line L1123 (-91.7186, -29.6999) -> (-91.6874, -29.9982)
  line L1124 (-91.7186, -29.6999) -> (-91.6874, -29.9983)
  line L1125 (-98.1515, -32.7016) -> (-97.9515, -32.7016)
  line L1126 (-97.9515, -32.7016) -> (-97.9515, -32.9516)
  line L1127 (-97.9515, -31.7016) -> (-98.1515, -31.7016)
  line L1128 (-97.9515, -31.5559) -> (-97.9515, -31.7016)
  line L1129 (-98.1515, -32.7016) -> (-98.1515, -31.7016)
  line L1130 (-96.0515, -32.9516) -> (-97.9515, -32.9516)
  line L1131 (-95.8515, -31.7016) -> (-95.8515, -32.7016)
  line L1132 (-96.0515, -32.9516) -> (-96.0515, -32.7016)
  line L1133 (-96.0515, -32.7016) -> (-95.8515, -32.7016)
  line L1134 (-95.8515, -31.7016) -> (-96.0515, -31.7016)
  line L1135 (-96.0515, -31.7016) -> (-96.0515, -31.5559)
  line L1136 (-97.7515, -31.7016) -> (-96.2515, -31.7016)
  line L1137 (-96.2515, -31.7016) -> (-96.2515, -32.7016)
  line L1138 (-96.2515, -32.7016) -> (-97.7515, -32.7016)
  line L1139 (-97.7515, -32.7016) -> (-97.7515, -31.7016)
  line L1140 (-96.4279, -31.8779) -> (-97.5752, -31.8779)
  line L1141 (-96.2515, -31.7016) -> (-96.4279, -31.8779)
  line L1142 (-97.7515, -31.7016) -> (-97.5752, -31.8779)
  line L1143 (-97.5752, -31.8779) -> (-97.5752, -32.5253)
  line L1144 (-97.7515, -32.7016) -> (-97.5752, -32.5253)
  line L1145 (-97.5752, -32.5253) -> (-96.4279, -32.5253)
  line L1146 (-96.2515, -32.7016) -> (-96.4279, -32.5253)
  line L1147 (-96.4279, -32.5253) -> (-96.4279, -31.8779)
  circle A26 centre (-97.2635, -32.2016) radius 0.1
  line L1148 (-97.1015, -32.3516) -> (-97.4254, -32.3516)
  line L1149 (-97.4254, -32.3516) -> (-97.4254, -32.0516)
  line L1150 (-97.4254, -32.0516) -> (-97.1015, -32.0516)
  line L1151 (-97.1015, -32.0516) -> (-97.1015, -32.3516)
  line L1152 (-98.1515, -33.9123) -> (-97.9515, -33.9123)
  line L1153 (-97.9515, -33.9123) -> (-97.9515, -34.1606)
  line L1154 (-98.1515, -33.9123) -> (-98.1515, -33.4516)
  line L1155 (-96.0515, -34.1606) -> (-97.9515, -34.1606)
  line L1156 (-95.8515, -33.4516) -> (-95.8515, -33.9123)
  line L1157 (-96.0515, -34.1606) -> (-96.0515, -33.9123)
  line L1158 (-96.0515, -33.9123) -> (-95.8515, -33.9123)
  line L1159 (-96.2515, -33.4516) -> (-96.2515, -33.9123)
  line L1160 (-96.2515, -33.9123) -> (-97.7515, -33.9123)
  line L1161 (-97.7515, -33.9123) -> (-97.7515, -33.4516)
  line L1162 (-97.5752, -33.4516) -> (-97.5752, -33.6212)
  line L1163 (-97.7515, -33.9123) -> (-97.5752, -33.6212)
  line L1164 (-97.5752, -33.6212) -> (-96.4279, -33.6212)
  line L1165 (-96.2515, -33.9123) -> (-96.4279, -33.6212)
  line L1166 (-96.4279, -33.6212) -> (-96.4279, -33.4516)
  line L1167 (-97.1015, -33.4719) -> (-97.4254, -33.4719)
  line L1168 (-97.4254, -33.4719) -> (-97.4254, -33.4516)
  line L1169 (-97.1015, -33.4516) -> (-97.1015, -33.4719)
  line L1170 (-105.4741, -21.298) -> (-105.4973, -21.4966)
  line L1171 (-105.4742, -21.2981) -> (-105.4741, -21.298)
  line L1172 (-105.7456, -21.4676) -> (-105.7457, -21.4677)
  line L1173 (-105.4973, -21.4966) -> (-105.7456, -21.4676)
  line L1174 (-105.7134, -23.5857) -> (-105.7411, -23.5825)
  line L1175 (-105.9662, -23.3549) -> (-105.7457, -21.4677)
  line L1176 (-105.4741, -21.298) -> (-105.2141, -21.3284)
  line L1177 (-104.2713, -21.7751) -> (-104.4762, -23.5289)
  line L1178 (-105.9661, -23.3548) -> (-105.7456, -21.4676)
  line L1179 (-104.7477, -23.6985) -> (-105.741, -23.5825)
  line L1180 (-105.7411, -23.5825) -> (-105.7298, -23.4858)
  line L1181 (-105.7458, -23.3806) -> (-105.9662, -23.3549)
  line L1182 (-105.9661, -23.3548) -> (-105.7178, -23.3838)
  line L1183 (-105.7178, -23.3838) -> (-105.741, -23.5825)
  line L1184 (-105.741, -23.5825) -> (-105.7411, -23.5825)
  line L1185 (-105.7178, -23.3838) -> (-105.7179, -23.3839)
  line L1186 (-105.9662, -23.3549) -> (-105.9661, -23.3548)
  line L1187 (-104.4762, -23.5289) -> (-104.4763, -23.5289)
  line L1188 (-104.7477, -23.6985) -> (-104.7245, -23.4999)
  line L1189 (-104.7245, -23.4999) -> (-104.4762, -23.5289)
  line L1190 (-104.7479, -23.6986) -> (-104.7477, -23.6985)
  line L1191 (-104.5272, -21.8113) -> (-104.7013, -23.3012)
  line L1192 (-104.7013, -23.3012) -> (-105.6945, -23.1852)
  line L1193 (-105.6945, -23.1852) -> (-105.5205, -21.6953)
  line L1194 (-105.5205, -21.6953) -> (-104.5272, -21.8113)
  line L1195 (-104.8561, -23.1057) -> (-104.7229, -21.9661)
  line L1196 (-104.7013, -23.3012) -> (-104.8561, -23.1057)
  line L1197 (-104.5272, -21.8113) -> (-104.7229, -21.9661)
  line L1198 (-104.7229, -21.9661) -> (-105.3659, -21.8909)
  line L1199 (-105.5205, -21.6953) -> (-105.3659, -21.8909)
  line L1200 (-105.3659, -21.8909) -> (-105.4991, -23.0305)
  line L1201 (-105.6945, -23.1852) -> (-105.4991, -23.0305)
  line L1202 (-105.4991, -23.0305) -> (-104.8561, -23.1057)
  circle A27 centre (-105.0806, -22.2381) radius 0.1
  line L1203 (-105.2484, -22.3816) -> (-105.2108, -22.0599)
  line L1204 (-105.2108, -22.0599) -> (-105.2108, -22.0599)
  line L1205 (-105.2484, -22.3816) -> (-105.2108, -22.0599)
  line L1206 (-105.2484, -22.3816) -> (-105.2484, -22.3816)
  line L1207 (-105.2108, -22.0599) -> (-104.9128, -22.0947)
  line L1208 (-104.9128, -22.0947) -> (-104.9504, -22.4164)
  line L1209 (-104.9504, -22.4164) -> (-104.9504, -22.4164)
  line L1210 (-104.9504, -22.4164) -> (-105.2484, -22.3816)
  line L1211 (-104.9504, -22.4164) -> (-105.2484, -22.3816)
  line L1212 (-104.239, -32.1396) -> (-104.4376, -32.1164)
  line L1213 (-104.2388, -32.1396) -> (-104.239, -32.1396)
  line L1214 (-104.4375, -32.1164) -> (-104.2388, -32.1396)
  line L1215 (-104.4376, -32.1164) -> (-104.4375, -32.1164)
  line L1216 (-104.268, -32.388) -> (-104.239, -32.1396)
  line L1217 (-104.2679, -32.3879) -> (-104.268, -32.388)
  line L1218 (-104.2388, -32.1396) -> (-104.2679, -32.3879)
  line L1219 (-104.1229, -31.1463) -> (-104.0963, -30.918)
  line L1220 (-104.3215, -31.1231) -> (-104.3216, -31.1232)
  line L1221 (-104.1228, -31.1463) -> (-104.3215, -31.1231)
  line L1222 (-104.0938, -30.898) -> (-104.1228, -31.1463)
  line L1223 (-104.0939, -30.8981) -> (-104.0938, -30.898)
  line L1224 (-104.4376, -32.1164) -> (-104.3216, -31.1232)
  line L1225 (-102.3808, -32.6084) -> (-104.268, -32.388)
  line L1226 (-104.4375, -32.1164) -> (-104.3215, -31.1231)
  line L1227 (-104.0938, -30.898) -> (-102.2066, -31.1185)
  line L1228 (-102.3807, -32.6084) -> (-104.2679, -32.3879)
  line L1229 (-102.037, -31.39) -> (-102.153, -32.3833)
  line L1230 (-102.1532, -32.3833) -> (-102.3517, -32.3602)
  line L1231 (-102.3807, -32.6084) -> (-102.3517, -32.3601)
  line L1232 (-102.3517, -32.3601) -> (-102.153, -32.3833)
  line L1233 (-102.153, -32.3833) -> (-102.1532, -32.3833)
  line L1234 (-102.3808, -32.6084) -> (-102.3807, -32.6084)
  line L1235 (-102.037, -31.39) -> (-102.2356, -31.3668)
  line L1236 (-102.2356, -31.3668) -> (-102.2066, -31.1185)
  line L1237 (-103.9242, -31.1696) -> (-102.4343, -31.3436)
  line L1238 (-102.4343, -31.3436) -> (-102.5503, -32.3369)
  line L1239 (-102.5503, -32.3369) -> (-104.0402, -32.1628)
  line L1240 (-104.0402, -32.1628) -> (-103.9242, -31.1696)
  line L1241 (-102.63, -31.4983) -> (-103.7696, -31.3652)
  line L1242 (-102.4343, -31.3436) -> (-102.63, -31.4983)
  line L1243 (-103.9242, -31.1696) -> (-103.7696, -31.3652)
  line L1244 (-103.7696, -31.3652) -> (-103.8447, -32.0082)
  line L1245 (-104.0402, -32.1628) -> (-103.8447, -32.0082)
  line L1246 (-103.8447, -32.0082) -> (-102.7051, -32.1413)
  line L1247 (-102.5503, -32.3369) -> (-102.7051, -32.1413)
  line L1248 (-102.7051, -32.1413) -> (-102.63, -31.4983)
  circle A28 centre (-103.4975, -31.7228) radius 0.1
  line L1249 (-103.3541, -31.8906) -> (-103.6757, -31.853)
  line L1250 (-103.6757, -31.8531) -> (-103.6757, -31.853)
  line L1251 (-103.3541, -31.8906) -> (-103.6757, -31.8531)
  line L1252 (-103.3541, -31.8906) -> (-103.3541, -31.8906)
  line L1253 (-103.6757, -31.853) -> (-103.6409, -31.5551)
  line L1254 (-103.6409, -31.5551) -> (-103.6409, -31.5551)
  line L1255 (-103.6757, -31.8531) -> (-103.6409, -31.5551)
  line L1256 (-103.6409, -31.5551) -> (-103.3192, -31.5927)
  line L1257 (-103.3192, -31.5927) -> (-103.3541, -31.8906)
  line L1258 (-100.4365, -20.0364) -> (-100.4365, -20.235)
  line L1259 (-100.4365, -20.235) -> (-100.6865, -20.235)
  line L1260 (-99.4365, -20.235) -> (-99.4365, -20.0364)
  line L1261 (-99.1865, -20.235) -> (-99.4365, -20.235)
  line L1262 (-99.1865, -22.2845) -> (-99.4365, -22.2845)
  line L1263 (-99.1865, -22.1222) -> (-99.1865, -22.2845)
  line L1264 (-99.4365, -22.3209) -> (-99.4365, -22.1222)
  line L1265 (-99.4365, -22.1222) -> (-99.1865, -22.1222)
  line L1266 (-99.4365, -22.4832) -> (-99.4365, -22.3209)
  line L1267 (-99.4365, -22.4832) -> (-100.4365, -22.4832)
  line L1268 (-100.4365, -20.0364) -> (-99.4365, -20.0364)
  line L1269 (-99.1865, -20.235) -> (-99.1865, -22.1222)
  line L1270 (-100.6865, -22.1222) -> (-100.6865, -20.235)
  line L1271 (-99.4365, -22.3209) -> (-100.4365, -22.3209)
  line L1272 (-100.4365, -22.2845) -> (-100.6865, -22.2845)
  line L1273 (-100.6865, -22.1222) -> (-100.4365, -22.1222)
  line L1274 (-100.4365, -22.1222) -> (-100.4365, -22.3209)
  line L1275 (-100.4365, -22.3209) -> (-100.4365, -22.4832)
  line L1276 (-100.6865, -22.2845) -> (-100.6865, -22.1222)
  line L1277 (-99.4365, -20.4337) -> (-99.4365, -21.9236)
  line L1278 (-99.4365, -21.9236) -> (-100.4365, -21.9236)
  line L1279 (-100.4365, -21.9236) -> (-100.4365, -20.4337)
  line L1280 (-100.4365, -20.4337) -> (-99.4365, -20.4337)
  line L1281 (-99.6129, -21.8644) -> (-99.6129, -20.7247)
  line L1282 (-99.4365, -21.9236) -> (-99.6129, -21.8644)
  line L1283 (-99.4365, -20.4337) -> (-99.6129, -20.7247)
  line L1284 (-99.6129, -20.7247) -> (-100.2602, -20.7247)
  line L1285 (-100.4365, -20.4337) -> (-100.2602, -20.7247)
  line L1286 (-100.2602, -20.7247) -> (-100.2602, -21.8644)
  line L1287 (-100.4365, -21.9236) -> (-100.2602, -21.8644)
  line L1288 (-100.2602, -21.8644) -> (-99.6129, -21.8644)
  ellipse E653 centre (-99.9365, -21.0054) end of major axis (-99.8365, -21.0054) minor radius 0.0993
  ellipse E654 centre (-99.9365, -21.0112) end of major axis (-99.8365, -21.0112) minor radius 0.0993 (-100.0365, -21.0112) -> (-99.8365, -21.0112) ccw
  line L1289 (-100.0365, -21.0112) -> (-100.0365, -21.0054)
  line L1290 (-99.8365, -21.0112) -> (-99.8365, -21.0054)
  line L1291 (-100.0865, -21.172) -> (-100.0865, -20.8504)
  line L1292 (-100.0865, -21.1952) -> (-100.0865, -21.172)
  line L1293 (-100.0865, -20.8504) -> (-99.7865, -20.8504)
  line L1294 (-99.7865, -20.8504) -> (-99.7865, -21.172)
  line L1295 (-99.7865, -21.1952) -> (-99.7865, -21.172)
  line L1296 (-99.7865, -21.172) -> (-100.0865, -21.172)
  line L1297 (-99.7865, -21.1952) -> (-100.0865, -21.1952)
  line L1298 (-97.9515, -30.752) -> (-98.1515, -30.752)
  line L1299 (-98.1515, -30.5898) -> (-97.9515, -30.5898)
  line L1300 (-98.1515, -30.752) -> (-98.1515, -30.5898)
  line L1301 (-97.9515, -30.8381) -> (-97.9515, -31.0004)
  line L1302 (-97.9515, -30.5898) -> (-97.9515, -30.8381)
  line L1303 (-97.9515, -29.5965) -> (-98.1515, -29.5965)
  line L1304 (-97.9515, -29.3482) -> (-97.9515, -29.5965)
  line L1305 (-95.8515, -30.752) -> (-96.0515, -30.752)
  line L1306 (-96.0515, -30.8381) -> (-96.0515, -30.5898)
  line L1307 (-96.0515, -30.5898) -> (-95.8515, -30.5898)
  line L1308 (-95.8515, -30.5898) -> (-95.8515, -30.752)
  line L1309 (-96.0515, -31.0004) -> (-96.0515, -30.8381)
  line L1310 (-96.0515, -31.0004) -> (-97.9515, -31.0004)
  line L1311 (-98.1515, -30.5898) -> (-98.1515, -29.5965)
  line L1312 (-97.9515, -29.3482) -> (-96.0515, -29.3482)
  line L1313 (-96.0515, -30.8381) -> (-97.9515, -30.8381)
  line L1314 (-95.8515, -29.5965) -> (-95.8515, -30.5898)
  line L1315 (-95.8515, -29.5965) -> (-96.0515, -29.5965)
  line L1316 (-96.0515, -29.5965) -> (-96.0515, -29.3482)
  line L1317 (-97.7515, -29.5965) -> (-96.2515, -29.5965)
  line L1318 (-96.2515, -29.5965) -> (-96.2515, -30.5898)
  line L1319 (-96.2515, -30.5898) -> (-97.7515, -30.5898)
  line L1320 (-97.7515, -30.5898) -> (-97.7515, -29.5965)
  line L1321 (-96.4279, -29.8876) -> (-97.5752, -29.8876)
  line L1322 (-96.2515, -29.5965) -> (-96.4279, -29.8876)
  line L1323 (-97.7515, -29.5965) -> (-97.5752, -29.8876)
  line L1324 (-97.5752, -29.8876) -> (-97.5752, -30.5305)
  line L1325 (-97.7515, -30.5898) -> (-97.5752, -30.5305)
  line L1326 (-97.5752, -30.5305) -> (-96.4279, -30.5305)
  line L1327 (-96.2515, -30.5898) -> (-96.4279, -30.5305)
  line L1328 (-96.4279, -30.5305) -> (-96.4279, -29.8876)
  ellipse E655 centre (-97.2635, -30.1801) end of major axis (-97.1635, -30.1801) minor radius 0.0993
  ellipse E656 centre (-97.2635, -30.1859) end of major axis (-97.1635, -30.1859) minor radius 0.0993 (-97.3635, -30.1859) -> (-97.1635, -30.1859) ccw
  line L1329 (-97.3635, -30.1859) -> (-97.3635, -30.1801)
  line L1330 (-97.1635, -30.1859) -> (-97.1635, -30.1801)
  line L1331 (-97.1015, -30.3349) -> (-97.4254, -30.3349)
  line L1332 (-97.4254, -30.358) -> (-97.4254, -30.3349)
  line L1333 (-97.1015, -30.358) -> (-97.4254, -30.358)
  line L1334 (-97.1015, -30.358) -> (-97.1015, -30.3349)
  line L1335 (-97.4254, -30.3349) -> (-97.4254, -30.0369)
  line L1336 (-97.4254, -30.0369) -> (-97.1015, -30.0369)
  line L1337 (-97.1015, -30.0369) -> (-97.1015, -30.3349)
  line L1338 (-91.6514, -32.3602) -> (-91.8499, -32.3833)
  line L1339 (-91.85, -32.3833) -> (-91.6514, -32.3601)
  line L1340 (-91.8499, -32.3833) -> (-91.85, -32.3833)
  line L1341 (-91.6224, -32.6084) -> (-91.6222, -32.6084)
  line L1342 (-91.6514, -32.3601) -> (-91.6224, -32.6084)
  line L1343 (-91.7674, -31.3668) -> (-91.9661, -31.39)
  line L1344 (-91.7965, -31.1185) -> (-91.7674, -31.3668)
  line L1345 (-89.9068, -30.918) -> (-89.8801, -31.1463)
  line L1346 (-89.9093, -30.898) -> (-89.9092, -30.8981)
  line L1347 (-89.6816, -31.1231) -> (-89.8803, -31.1463)
  line L1348 (-89.8803, -31.1463) -> (-89.9093, -30.898)
  line L1349 (-89.6815, -31.1232) -> (-89.6816, -31.1231)
  line L1350 (-89.6815, -31.1232) -> (-89.5654, -32.1164)
  line L1351 (-89.7351, -32.388) -> (-91.6222, -32.6084)
  line L1352 (-91.85, -32.3833) -> (-91.9661, -31.39)
  line L1353 (-91.7965, -31.1185) -> (-89.9093, -30.898)
  line L1354 (-89.7352, -32.3879) -> (-91.6224, -32.6084)
  line L1355 (-89.6816, -31.1231) -> (-89.5656, -32.1164)
  line L1356 (-89.5654, -32.1164) -> (-89.7641, -32.1396)
  line L1357 (-89.7641, -32.1396) -> (-89.7351, -32.388)
  line L1358 (-89.7352, -32.3879) -> (-89.7642, -32.1396)
  line L1359 (-89.7642, -32.1396) -> (-89.5656, -32.1164)
  line L1360 (-89.5656, -32.1164) -> (-89.5654, -32.1164)
  line L1361 (-89.7642, -32.1396) -> (-89.7641, -32.1396)
  line L1362 (-89.7351, -32.388) -> (-89.7352, -32.3879)
  line L1363 (-91.5688, -31.3436) -> (-90.0789, -31.1696)
  line L1364 (-90.0789, -31.1696) -> (-89.9629, -32.1628)
  line L1365 (-89.9629, -32.1628) -> (-91.4527, -32.3369)
  line L1366 (-91.4527, -32.3369) -> (-91.5688, -31.3436)
  line L1367 (-90.2335, -31.3652) -> (-91.3731, -31.4983)
  line L1368 (-90.0789, -31.1696) -> (-90.2335, -31.3652)
  line L1369 (-91.5688, -31.3436) -> (-91.3731, -31.4983)
  line L1370 (-91.3731, -31.4983) -> (-91.298, -32.1413)
  line L1371 (-91.4527, -32.3369) -> (-91.298, -32.1413)
  line L1372 (-91.298, -32.1413) -> (-90.1584, -32.0082)
  line L1373 (-89.9629, -32.1628) -> (-90.1584, -32.0082)
  line L1374 (-90.1584, -32.0082) -> (-90.2335, -31.3652)
  circle A29 centre (-91.0259, -31.7836) radius 0.1
  line L1375 (-90.8477, -31.9138) -> (-91.1693, -31.9514)
  line L1376 (-91.1693, -31.9514) -> (-91.1693, -31.9514)
  line L1377 (-90.8477, -31.9138) -> (-91.1693, -31.9514)
  line L1378 (-90.8477, -31.9138) -> (-90.8477, -31.9138)
  line L1379 (-91.1693, -31.9514) -> (-91.2041, -31.6534)
  line L1380 (-91.2041, -31.6534) -> (-90.8825, -31.6159)
  line L1381 (-90.8825, -31.6159) -> (-90.8825, -31.6159)
  line L1382 (-90.8825, -31.6159) -> (-90.8477, -31.9138)
  line L1383 (-90.8825, -31.6159) -> (-90.8477, -31.9138)
  line L1384 (-104.1982, -17.698) -> (-104.1794, -17.4989)
  line L1385 (-104.1793, -17.4989) -> (-104.1981, -17.698)
  line L1386 (-104.1794, -17.4989) -> (-104.1793, -17.4989)
  line L1387 (-104.447, -17.6744) -> (-104.4471, -17.6744)
  line L1388 (-104.1981, -17.698) -> (-104.447, -17.6744)
  line L1389 (-103.2026, -17.7923) -> (-103.1837, -17.5932)
  line L1390 (-102.9537, -17.8159) -> (-103.2026, -17.7923)
  line L1391 (-104.468, -17.8945) -> (-104.4471, -17.6744)
  line L1392 (-104.1793, -17.4989) -> (-103.1837, -17.5932)
  line L1393 (-102.9537, -17.8159) -> (-103.133, -19.7075)
  line L1394 (-104.6131, -19.4267) -> (-104.447, -17.6744)
  line L1395 (-103.4008, -19.883) -> (-103.5532, -19.8685)
  line L1396 (-103.133, -19.7075) -> (-103.1331, -19.7075)
  line L1397 (-103.4008, -19.883) -> (-103.3819, -19.6839)
  line L1398 (-103.3819, -19.6839) -> (-103.133, -19.7075)
  line L1399 (-103.4009, -19.883) -> (-103.4008, -19.883)
  line L1400 (-103.2215, -17.9914) -> (-103.363, -19.4848)
  line L1401 (-103.363, -19.4848) -> (-104.3585, -19.3904)
  line L1402 (-104.3585, -19.3904) -> (-104.217, -17.8971)
  line L1403 (-104.217, -17.8971) -> (-103.2215, -17.9914)
  line L1404 (-103.522, -19.2926) -> (-103.4137, -18.1504)
  line L1405 (-103.363, -19.4848) -> (-103.522, -19.2926)
  line L1406 (-103.2215, -17.9914) -> (-103.4137, -18.1504)
  line L1407 (-103.4137, -18.1504) -> (-104.0582, -18.0893)
  line L1408 (-104.217, -17.8971) -> (-104.0582, -18.0893)
  line L1409 (-104.0582, -18.0893) -> (-104.1664, -19.2315)
  line L1410 (-104.3585, -19.3904) -> (-104.1664, -19.2315)
  line L1411 (-104.1664, -19.2315) -> (-103.522, -19.2926)
  circle A30 centre (-103.7653, -18.4302) radius 0.1
  line L1412 (-103.93, -18.5772) -> (-103.8994, -18.2548)
  line L1413 (-103.93, -18.5772) -> (-103.8994, -18.2548)
  line L1414 (-103.8994, -18.2548) -> (-103.6007, -18.2831)
  line L1415 (-103.6007, -18.2831) -> (-103.6313, -18.6055)
  line L1416 (-103.6313, -18.6055) -> (-103.93, -18.5772)
  line L1417 (-102.708, -28.311) -> (-102.7081, -28.311)